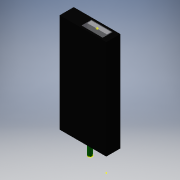
# Autodesk Inventor part: usbHubSmall
Saved by Autodesk Inventor 2016 (Build 200138000, 138)
## iProperties
Created: 2015-10-18
Part Number: usbHubSmall
Material: Generic
Document SubType Name: Modeling
Designer: Artur
Density: 1 g/cm^3
Appearance: Default
Mass: 20.1467 g
Surface Area: 105.182 cm^2
Volume: 20.1467 cm^3
Author: Artur
Autodesk Inventor part; units mm, degrees
ref_plane "YZ Plane" through (0, 0, 0) normal (1, 0, 0) x (0, 1, 0)
ref_plane "XZ Plane" through (0, 0, 0) normal (0, 1, 0) x (-1, 0, 0)
ref_plane "XY Plane" through (0, 0, 0) normal (0, 0, 1) x (1, 0, 0)
sketch "Sketch1" plane through (0, 0, 0) normal (0, 1, 0) x (-1, 0, 0)
  line L0 (0, 0) -> (33, 0)
  line L1 (33, 0) -> (33, -70)
  line L2 (33, -70) -> (0, -70)
  line L3 (0, -70) -> (0, 0)
  dimension "d0" = 70
  dimension "d1" = 33
  constraints: 8 end point, 2 parallel, 1 horizontal, 1 perpendicular
  measures "d0" distance of L0.end L1.end
  measures "d1" distance of L0.start L0.end
extrude "Extrusion1" add sketch "Sketch1" along normal blind 10
sketch "Sketch2" plane through (-33, 0, 0) normal (0, 0, 1) x (1, 0, 0)
  line L0 (14, 1.5) -> (29, 1.5)
  line L1 (14, 1.5) -> (14, 8.5)
  line L2 (14, 8.5) -> (29, 8.5)
  line L3 (29, 8.5) -> (29, 1.5)
  line L4 (14.5, 8) -> (28.5, 8)
  line L5 (28.5, 8) -> (28.5, 5)
  line L6 (28.5, 5) -> (14.5, 5)
  line L7 (14.5, 5) -> (14.5, 8)
  line L8 (33, 0) -> (33, 10) projected
  line L9 (33, 0) -> (0, 0) projected
  point P0 (21.5, 1.5)
  point P1 (30, -14)
  point P2 (21.5, 5)
  point P3 (30, -14)
  point P4 (30, -14)
  dimension "d4" = 15
  dimension "d5" = 7
  dimension "d6" = 14
  dimension "d7" = 3
  dimension "d8" = 0.5
  dimension "d9" = 0.5
  dimension "d22" = 4
  dimension "d23" = 1.5
  constraints: 16 end point, 3 perpendicular, 2 horizontal, 2 midpoint, 2 parallel, 1 vertical
  measures "d4" distance of L0.start L0.end
  measures "d5" distance of L0.start L1.end
  measures "d6" distance of L4.start L4.end
  measures "d7" distance of L6.end L4.start
  measures "d8" distance between parallel lines of L1 L7
  measures "d9" distance between parallel lines of L2 L4
  measures "d22" distance between parallel lines of L3 L8
  measures "d23" distance between parallel lines of L9 L0
extrude "Extrusion2" cut sketch "Sketch2" against normal blind 12
sketch "Sketch3" plane through (-33, 0, -70) normal (-1, 0, 0) x (0, 0, 1)
  line L0 (7, 1.5) -> (22, 1.5)
  line L1 (7, 1.5) -> (7, 8.5)
  line L2 (7, 8.5) -> (22, 8.5)
  line L3 (22, 8.5) -> (22, 1.5)
  line L4 (7.5, 8) -> (21.5, 8)
  line L5 (21.5, 8) -> (21.5, 5)
  line L6 (21.5, 5) -> (7.5, 5)
  line L7 (7.5, 5) -> (7.5, 8)
  line L8 (0, 0) -> (0, 10) projected
  line L9 (70, 0) -> (0, 0) projected
  line L10 (14.5, 8.5) -> (14.5, 1.5) construction
  line L11 (28, 1.5) -> (28, 8.5)
  line L12 (28.5, 5) -> (28.5, 8)
  line L13 (28.5, 8) -> (42.5, 8)
  line L14 (42.5, 8) -> (42.5, 5)
  line L15 (42.5, 5) -> (28.5, 5)
  line L16 (28, 1.5) -> (43, 1.5)
  line L17 (28, 8.5) -> (43, 8.5)
  line L18 (43, 8.5) -> (43, 1.5)
  line L19 (35.5, 8.5) -> (35.5, 1.5) construction
  line L20 (49, 1.5) -> (49, 8.5)
  line L21 (49.5, 5) -> (49.5, 8)
  line L22 (49.5, 8) -> (63.5, 8)
  line L23 (63.5, 8) -> (63.5, 5)
  line L24 (63.5, 5) -> (49.5, 5)
  line L25 (49, 1.5) -> (64, 1.5)
  line L26 (49, 8.5) -> (64, 8.5)
  line L27 (64, 8.5) -> (64, 1.5)
  line L28 (56.5, 8.5) -> (56.5, 1.5) construction
  point P0 (14.5, 5)
  point P1 (35.5, 5)
  point P2 (56.5, 5)
  dimension "d26" = 15
  dimension "d27" = 7
  dimension "d28" = 14
  dimension "d29" = 3
  dimension "d30" = 0.5
  dimension "d31" = 0.5
  dimension "d32" = 7
  dimension "d33" = 1.5
  dimension "d36" = 21
  constraints: 54 end point, 3 horizontal, 3 midpoint, 3 perpendicular, 2 parallel, 1 collinear, 1 vertical, 39 other
  measures "d26" distance of L1.start L0.end
  measures "d27" distance of L1.start L1.end
  measures "d28" distance of L7.end L4.end
  measures "d29" distance of L7.start L7.end
  measures "d30" distance between parallel lines of L1 L7
  measures "d31" distance between parallel lines of L2 L4
  measures "d32" distance between parallel lines of L8 L1
  measures "d33" distance from line of L9 L1.start
  measures "d36" distance of L1.start L11.start
extrude "Extrusion3" cut sketch "Sketch3" against normal blind 12
sketch "Sketch4" plane through (0, 0, -70) normal (0, 0, -1) x (-1, 0, 0)
  circle A0 centre (16.5, 5) radius 1.5
  line L0 (33, 0) -> (0, 0) projected
  line L1 (0, 10) -> (33, 10) projected
  line L2 (0, 0) -> (0, 10) projected
  line L3 (33, 0) -> (33, 10) projected
  dimension "d43" = 3
  dimension "d44" = 10
  dimension "d45" = 33
  dimension "d46" = 5
  dimension "d47" = 16.5
  constraints: 1 centre point
  measures "d43" diameter of A0
  measures "d44" distance between parallel lines of L0 L1
  measures "d45" distance between parallel lines of L2 L3
  measures "d46" distance from line of L0 A0.centre
  measures "d47" distance from line of L3 A0.centre
extrude "Extrusion4" add sketch "Sketch4" along normal blind 10 contours A0
sketch "Sketch5" plane through (-16.5, 5, -80) normal (0, 0, -1) x (-1, 0, 0)
  circle A0 centre (0, 0) radius 1.5 projected
  point P0 (-16.5, -5)
  constraints: 1 coincident
equation "\"d46\" = 0.5 * d44"
equation "\"d47\" = 0.5 * d45"
body "Solid1"
